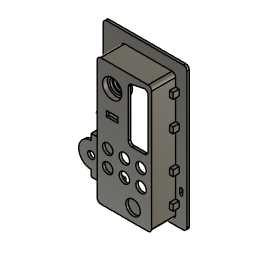
WIP-KV-1375DInputPanel-MULTIMOD (Autodesk Fusion 360 design; units mm, degrees)
Autodesk Fusion 360 part; units mm, degrees
sketch "Body" plane through (0, 0, 0) normal (0, 1, 0) x (1, 0, 0)
  line L0 (60.5, -7.2844) -> (60.5, -107.2844)
  circle A0 centre (0, -25.75) radius 10.5
  circle A1 centre (0, -25.75) radius 3
  arc A2 (18, -4.2844) -> (15, -7.2844) centre (18, -7.2844) ccw
  arc A3 (67, -119.5) -> (70, -116.5) centre (67, -116.5) ccw
  circle A4 centre (5.375, -59) radius 1
  line L1 (15, -4.2844) -> (19, -4.2844) construction
  line L2 (58.5105, -108.25) -> (17.001, -108.25)
  circle A5 centre (9.2756, -62.8749) radius 1
  arc A6 (57.5, -110.2844) -> (60.5, -107.2844) centre (57.5, -107.2844) ccw
  line L3 (0, -10) -> (0, -3)
  line L4 (15, -41.5) -> (0, -41.5)
  line L5 (15, -10) -> (15, -41.5)
  circle A7 centre (9.25, -59) radius 1.2
  arc A8 (15, -107.2844) -> (18, -110.2844) centre (18, -107.2844) ccw
  line L6 (70, -3) -> (70, -116.5)
  arc A9 (60.5, -7.2844) -> (57.5, -4.2844) centre (57.5, -7.2844) ccw
  line L7 (15, -107.2844) -> (15, -7.2844)
  arc A10 (70, -3) -> (67, 0) centre (67, -3) ccw
  circle A11 centre (9.25, -59) radius 3.875
  line L8 (17.0105, -6.25) -> (58.5105, -6.25)
  line L9 (18, -4.2844) -> (57.5, -4.2844)
  line L10 (0, -10) -> (15, -10)
  line L11 (3, 0) -> (67, 0)
  line L12 (67, -119.5) -> (3, -119.5)
  line L13 (57.5, -110.2844) -> (18, -110.2844)
  line L14 (58.5105, -6.25) -> (58.5105, -108.25)
  line L15 (0, -116.5) -> (0, -10)
  arc A12 (3, 0) -> (0, -3) centre (3, -3) ccw
  line L16 (15, -59) -> (9.25, -59)
  arc A13 (0, -116.5) -> (3, -119.5) centre (3, -116.5) ccw
  circle A14 centre (9.25, -55.125) radius 1
  line L17 (15, -100.2844) -> (12, -100.2844)
  line L18 (12, -100.2844) -> (12, -95.25)
  line L19 (12, -95.25) -> (15, -95.25)
  line L20 (15, -95.25) -> (15, -100.2844)
  line L21 (60.5, -100.2844) -> (63.5, -100.2844)
  line L22 (63.5, -100.2844) -> (63.5, -95.25)
  line L23 (63.5, -95.25) -> (60.5, -95.25)
  line L24 (60.5, -95.25) -> (60.5, -100.2844)
  line L25 (60.5, -75.25) -> (63.5, -75.25)
  line L26 (63.5, -75.25) -> (63.5, -70.25)
  line L27 (63.5, -70.25) -> (60.5, -70.25)
  line L28 (60.5, -70.25) -> (60.5, -75.25)
  line L29 (60.5, -44.25) -> (63.5, -44.25)
  line L30 (63.5, -44.25) -> (63.5, -39.25)
  line L31 (63.5, -39.25) -> (60.5, -39.25)
  line L32 (60.5, -39.25) -> (60.5, -44.25)
  line L33 (60.5, -14.2844) -> (63.5, -14.2844)
  line L34 (63.5, -14.2844) -> (63.5, -19.25)
  line L35 (63.5, -19.25) -> (60.5, -19.25)
  line L36 (60.5, -19.25) -> (60.5, -14.2844)
  line L37 (12.925, -58) -> (15, -58)
  line L38 (15, -58) -> (15, -60)
  line L39 (15, -60) -> (12.925, -60)
  line L40 (12.925, -60) -> (12.925, -58)
  line L41 (17.001, -108.25) -> (17.0105, -6.25)
  circle A15 centre (65.25, -28.5) radius 1.25
  circle A16 centre (65.25, -25) radius 1.25
  line L42 (65.25, -28.5) -> (64, -28.5)
  line L43 (65.25, -25) -> (66.5, -25)
  line L44 (64, -28.5) -> (66.5, -28.5)
  line L45 (66.5, -28.5) -> (66.5, -25)
  line L46 (66.5, -25) -> (64, -25)
  line L47 (64, -25) -> (64, -28.5)
  line L48 (15, -12) -> (0, -12)
  line L49 (15, -39.5) -> (0, -39.5)
  line L50 (15, -10) -> (17.0101, -10.0002)
  line L51 (15, -12) -> (17.0099, -12.0002)
  line L52 (15, -39.5) -> (17.0074, -39.5002)
  line L53 (15, -41.5) -> (17.0072, -41.5002)
  point P0 (54.389, -114.7651)
  point P1 (37.889, -114.7651)
  point P2 (70, 0)
  point P3 (0, -119.5)
  point P4 (60.5, -4.2844)
  point P5 (15, -110.2844)
  dimension "d245" = 70
  dimension "d246" = 119.5
  dimension "d247" = 45.5
  dimension "d248" = 106
  dimension "d249" = 31.5
  dimension "d250" = 21
  dimension "d251" = 6
  dimension "d252" = 5.75
  dimension "d253" = 2.4
  dimension "d254" = 7.75
  dimension "d256" = 2
  dimension "d257" = 2
  dimension "d258" = 2
  dimension "d260" = 41.5
  dimension "d261" = 102
  dimension "d262" = 3
  dimension "d263" = 3
  dimension "d484" = 10
  dimension "d485" = 10
  dimension "d486" = 10
  dimension "d487" = 20
  dimension "d488" = 20
  dimension "d757" = 2.5
  dimension "d758" = 2.5
  constraint horizontal L11
  constraint vertical L6
  constraint horizontal L12
  constraint horizontal L9
  constraint vertical L0
  constraint horizontal L13
  constraint vertical L7
  constraint horizontal L4
  constraint horizontal L10
  constraint vertical L5
  constraint coincident L4.start L7
  constraint concentric A0 A1
  constraint coincident L16.start L7
  constraint perpendicular L7 L16
  constraint coincident A7.centre A11.centre
  constraint coincident A5.centre A11
  constraint coincident A4.centre A11
  constraint coincident A14.centre A11
  constraint horizontal L1
  constraint horizontal L8
  constraint vertical L14
  constraint horizontal L2
  constraint perpendicular L10 L15
  constraint coincident L48.end L15
  constraint coincident L49.end L15
  constraint perpendicular L3 L11
  constraint coincident P3 L12
  constraint coincident P3 L15
  constraint tangent L12 A13
  constraint tangent L15 A13
  constraint tangent A3 L6
  constraint tangent A3 L12
  constraint equal A3 A13
  constraint coincident P2 L11
  constraint coincident P2 L6
  constraint tangent A10 L11
  constraint tangent L6 A10
  constraint equal A10 A13
  constraint coincident origin L11
  constraint tangent L3 A12
  constraint tangent L11 A12
  constraint equal A12 A13
  constraint coincident P5 L13
  constraint coincident P5 L7
  constraint tangent A8 L13
  constraint tangent A8 L7
  constraint tangent L0 A6
  constraint tangent A6 L13
  constraint equal A6 A8
  constraint coincident P4 L9
  constraint coincident P4 L0
  constraint tangent A9 L9
  constraint tangent L0 A9
  constraint equal A8 A9
  constraint coincident L1.start L7
  constraint coincident L1.start L9
  constraint tangent A2 L7
  constraint tangent A2 L9
  constraint equal A2 A8
  constraint horizontal L17
  constraint vertical L18
  constraint horizontal L19
  constraint vertical L20
  constraint coincident L7 L17.start
  constraint horizontal L21
  constraint vertical L22
  constraint horizontal L23
  constraint vertical L24
  constraint coincident L0 L21.start
  constraint horizontal L25
  constraint vertical L26
  constraint horizontal L27
  constraint vertical L28
  constraint coincident L0 L25.start
  constraint horizontal L29
  constraint vertical L30
  constraint horizontal L31
  constraint vertical L32
  constraint coincident L0 L29.start
  constraint horizontal L33
  constraint vertical L34
  constraint horizontal L35
  constraint vertical L36
  constraint coincident L0 L33.start
  constraint horizontal L37
  constraint vertical L38
  constraint horizontal L39
  constraint vertical L40
  constraint coincident L7 L38.end
  constraint coincident A15.centre L42.start
  constraint coincident A15 L42.end
  constraint horizontal L42
  constraint coincident A16.centre L43.start
  constraint coincident A16 L43.end
  constraint horizontal L43
  constraint horizontal L44
  constraint vertical L45
  constraint horizontal L46
  constraint vertical L47
  constraint coincident L5 L48.start
  constraint coincident L5 L49.start
  constraint coincident L41 L50.end
  constraint perpendicular L41 L50
  constraint coincident L41 L51.end
  constraint perpendicular L41 L51
  constraint coincident L41 L52.end
  constraint perpendicular L41 L52
  constraint coincident L41 L53.end
  constraint perpendicular L41 L53
  measures "d245" distance of origin P2
  measures "d246" distance of origin P3
  measures "d247" distance of L1.start P4
  measures "d248" distance of L1.start P5
  measures "d249" distance of L5.start L4.start
  measures "d250" diameter of A0
  measures "d251" diameter of A1
  measures "d252" distance of L16.start A7.centre
  measures "d253" diameter of A7
  measures "d254" diameter of A11
  measures "d256" diameter of A5
  measures "d257" diameter of A4
  measures "d258" diameter of A14
  measures "d260" distance of L8.start L8.end
  measures "d261" distance of L8.start L2.end
  measures "d262" radius of A13
  measures "d263" radius of A8
  measures "d484" distance of L13 L21
  measures "d485" distance of L9 L33
  measures "d486" distance of L13 L17
  measures "d487" distance of L31 L35
  measures "d488" distance of L23 L25
  measures "d757" diameter of A15
  measures "d758" diameter of A16
sketch "SCART" plane through (0, 0, 0) normal (0, 1, 0) x (1, 0, 0)
  line L0 (53.8762, -105.9949) -> (43.3762, -103.763)
  arc A0 (41, -100.8286) -> (43.3762, -103.763) centre (44, -100.8286) ccw
  arc A1 (53.8762, -105.9949) -> (57.5, -103.0604) centre (54.5, -103.0604) ccw
  arc A2 (44, -58.6151) -> (41, -61.6151) centre (44, -61.6151) ccw
  arc A3 (57.5, -61.6151) -> (54.5, -58.6151) centre (54.5, -61.6151) ccw
  line L1 (44, -56.6151) -> (55.389, -56.6151)
  line L2 (59.889, -61.6151) -> (59.889, -109.0604)
  line L3 (59.889, -109.0604) -> (39, -109.0604)
  line L4 (39, -109.0604) -> (39, -61.6151)
  arc A4 (44, -56.6151) -> (39, -61.6151) centre (44, -61.6151) ccw
  line L5 (59.889, -61.6151) -> (59.889, -56.6151)
  line L6 (59.889, -56.6151) -> (55.389, -56.6151)
  line L7 (41, -100.8286) -> (41, -61.6151)
  line L8 (44, -58.6151) -> (54.5, -58.6151)
  line L9 (57.5, -61.6151) -> (57.5, -103.0604)
  dimension "d178" = 3
  dimension "d179" = 3
  dimension "d180" = 3
  dimension "d181" = 3
  dimension "d183" = 39.2135
  constraint tangent L0 A1
  constraint tangent L0 A0
  constraint horizontal L1
  constraint vertical L2
  constraint horizontal L3
  constraint vertical L4
  constraint tangent L1 A4
  constraint tangent L4 A4
  constraint perpendicular L1 L5
  constraint perpendicular L5 L6
  constraint tangent A2 L7
  constraint tangent A3 L8
  constraint tangent A1 L9
  measures "d178" radius of A1
  measures "d179" radius of A0
  measures "d180" radius of A2
  measures "d181" radius of A3
  measures "d183" distance of A2.end A0.start
sketch "Components" plane through (0, 0, 0) normal (0, 1, 0) x (1, 0, 0)
  circle A0 centre (37.705, -33.2295) radius 5.75
  circle A1 centre (37.705, -33.2295) radius 6.5
  circle A2 centre (23.805, -33.2295) radius 6.5
  circle A3 centre (23.805, -33.2295) radius 5.75
  circle A4 centre (51.605, -33.2295) radius 5.75
  circle A5 centre (51.605, -33.2295) radius 6.5
  circle A6 centre (37.705, -33.2295) radius 4.375
  circle A7 centre (23.805, -33.2295) radius 4.375
  circle A8 centre (51.605, -33.2295) radius 4.375
  circle A9 centre (51.605, -47.1295) radius 6.5
  circle A10 centre (37.705, -47.1295) radius 5.75
  circle A11 centre (51.605, -47.1295) radius 5.75
  circle A12 centre (37.705, -47.1295) radius 6.5
  circle A13 centre (23.805, -47.1295) radius 5.75
  circle A14 centre (37.705, -47.1295) radius 4.375
  circle A15 centre (51.605, -47.1295) radius 4.375
  circle A16 centre (23.805, -47.1295) radius 6.5
  circle A17 centre (23.805, -47.1295) radius 4.375
  circle A18 centre (27.5005, -92.5463) radius 4.825
  circle A19 centre (27.5005, -92.5463) radius 9
  circle A20 centre (27.5005, -92.5463) radius 8
  line L0 (19.5004, -75.9605) -> (35.5004, -75.9605)
  line L1 (22.7504, -74.4605) -> (22.7504, -69.9605)
  line L2 (19.5004, -68.4605) -> (19.5004, -75.9605)
  line L3 (32.2504, -69.9605) -> (32.2504, -74.4605)
  line L4 (22.7504, -69.9605) -> (32.2504, -69.9605)
  line L5 (32.2504, -74.4605) -> (22.7504, -74.4605)
  line L6 (33.2504, -75.4605) -> (33.2504, -68.9605)
  line L7 (21.7504, -68.9605) -> (21.7504, -75.4605)
  line L8 (33.2504, -68.9605) -> (21.7504, -68.9605)
  line L9 (35.5004, -68.4605) -> (19.5004, -68.4605)
  line L10 (15.5004, -77.9605) -> (15.5004, -66.4605)
  line L11 (38.5004, -66.4605) -> (38.5004, -77.9605)
  line L12 (35.5004, -75.9605) -> (35.5004, -68.4605)
  line L13 (21.7504, -75.4605) -> (33.2504, -75.4605)
  line L14 (15.5004, -66.4605) -> (38.5004, -66.4605)
  line L15 (38.5004, -77.9605) -> (15.5004, -77.9605)
  circle A21 centre (55.0033, -15.1761) radius 1.25
  circle A22 centre (35.0033, -15.1761) radius 1.25
  circle A23 centre (45.0033, -15.1761) radius 6.125
  line L16 (21.9579, -89.347) -> (21.958, -95.747)
  line L17 (27.5008, -98.9466) -> (33.0434, -95.7468)
  line L18 (27.5003, -86.1467) -> (21.9579, -89.347)
  line L19 (33.0434, -95.7468) -> (33.0428, -89.3468)
  line L20 (33.0428, -89.3468) -> (27.5003, -86.1467)
  line L21 (21.958, -95.747) -> (27.5008, -98.9466)
  line L22 (51.605, -47.1295) -> (51.605, -33.2295)
  line L23 (23.805, -33.2295) -> (23.805, -47.1295)
  line L24 (37.705, -47.1295) -> (37.705, -33.2295)
  line L25 (23.805, -47.1295) -> (37.705, -47.1295)
  line L26 (37.705, -47.1295) -> (51.605, -47.1295)
  line L27 (30.755, -47.1295) -> (30.755, -33.7)
  line L28 (44.655, -47.1295) -> (44.655, -33.7)
  circle A24 centre (30.755, -40.1795) radius 1.25
  circle A25 centre (44.655, -40.1795) radius 1.25
  circle A26 centre (55.0033, -15.1761) radius 2.93
  circle A27 centre (35.0033, -15.1761) radius 2.9
  circle A28 centre (45.0033, -15.1761) radius 6.85
  line L29 (56.0709, -17.9047) -> (48.0733, -21.2996)
  line L30 (56.0709, -12.4476) -> (48.0733, -9.0526)
  line L31 (34.0209, -17.9047) -> (41.9332, -21.2996)
  line L32 (34.0209, -12.4476) -> (41.9332, -9.0526)
  circle A29 centre (27.5005, -92.5463) radius 6
  line L33 (24.6242, -97.8165) -> (30.3742, -97.8165)
  line L34 (44.655, -33.7) -> (45.1221, -33.7)
  line L35 (44.655, -33.7) -> (44.188, -33.7)
  line L36 (30.755, -33.7) -> (31.2221, -33.7)
  line L37 (30.755, -33.7) -> (30.288, -33.7)
  point P0 (37.889, -53.1151)
  point P1 (27.5005, -92.5463)
  dimension "d301" = 8.75
  dimension "d302" = 8.75
  dimension "d303" = 8.75
  dimension "d304" = 11.5
  dimension "d305" = 11.5
  dimension "d306" = 11.5
  dimension "d307" = 13
  dimension "d308" = 13
  dimension "d309" = 13
  dimension "d334" = 13.9
  dimension "d384" = 8.75
  dimension "d385" = 8.75
  dimension "d386" = 8.75
  dimension "d387" = 11.5
  dimension "d388" = 11.5
  dimension "d389" = 11.5
  dimension "d390" = 13
  dimension "d391" = 13
  dimension "d392" = 13
  dimension "d393" = 13.9
  dimension "d395" = 13.9
  dimension "d400" = 9.65
  dimension "d401" = 16
  dimension "d402" = 18
  dimension "d403" = 7.5
  dimension "d404" = 16
  dimension "d405" = 4.5
  dimension "d406" = 9.5
  dimension "d407" = 6.5
  dimension "d408" = 11.5
  dimension "d409" = 7.5
  dimension "d410" = 16
  dimension "d411" = 11.5
  dimension "d412" = 6.5
  dimension "d413" = 4.5
  dimension "d414" = 2.25
  dimension "d415" = 2.25
  dimension "d416" = 1
  dimension "d417" = 12.25
  dimension "d420" = 2.5
  dimension "d422" = 2.5
  dimension "d787" = 13.9
  dimension "d788" = 13.9
  dimension "d791" = 2.5
  dimension "d792" = 2.5
  dimension "d793" = 13.9
  dimension "d805" = 5.86
  dimension "d806" = 5.8
  dimension "d807" = 13.7
  dimension "d818" = 3
  dimension "d851" = 12
  dimension "d852" = 5.75
  constraint concentric A3 A7
  constraint concentric A0 A6
  constraint concentric A4 A8
  constraint concentric A2 A3
  constraint concentric A1 A6
  constraint concentric A5 A8
  constraint concentric A13 A17
  constraint concentric A10 A14
  constraint concentric A11 A15
  constraint concentric A13 A16
  constraint concentric A12 A14
  constraint concentric A9 A15
  constraint concentric A18 A20
  constraint concentric A18 A19
  constraint perpendicular L1 L4
  constraint perpendicular L7 L8
  constraint perpendicular L2 L9
  constraint perpendicular L0 L12
  constraint perpendicular L3 L5
  constraint horizontal L15
  constraint vertical L10
  constraint horizontal L14
  constraint vertical L11
  constraint vertical L22
  constraint vertical L23
  constraint coincident A4.centre A5.centre
  constraint coincident A13.centre A16.centre
  constraint coincident A10.centre A12.centre
  constraint coincident A0.centre A1.centre
  constraint perpendicular L24 L25
  constraint coincident A9.centre A11.centre
  constraint perpendicular L22 L26
  constraint midpoint L25 L27.start
  constraint perpendicular L25 L27
  constraint midpoint L26 L28.start
  constraint perpendicular L26 L28
  constraint coincident L27 A24.centre
  constraint coincident L28 A25.centre
  constraint concentric A21 A26
  constraint concentric A22 A27
  constraint coincident A26 L29.start
  constraint coincident A28 L29.end
  constraint coincident A26 L30.start
  constraint coincident A28 L30.end
  constraint coincident A28 L32.end
  constraint coincident A28 L31.end
  constraint coincident A27 L31.start
  constraint coincident A27 L32.start
  constraint coincident P1 A18.centre
  constraint horizontal L33
  constraint coincident A5 L34.end
  constraint perpendicular L28 L34
  constraint coincident A1 L35.end
  constraint perpendicular L28 L35
  constraint coincident A1 L36.end
  constraint perpendicular L27 L36
  constraint coincident A2 L37.end
  constraint perpendicular L27 L37
  measures "d301" diameter of A7
  measures "d302" diameter of A6
  measures "d303" diameter of A8
  measures "d304" diameter of A3
  measures "d305" diameter of A0
  measures "d306" diameter of A4
  measures "d307" diameter of A2
  measures "d308" diameter of A1
  measures "d309" diameter of A5
  measures "d334" distance of A4.centre A0.centre
  measures "d384" diameter of A17
  measures "d385" diameter of A14
  measures "d386" diameter of A15
  measures "d387" diameter of A13
  measures "d388" diameter of A10
  measures "d389" diameter of A11
  measures "d390" diameter of A16
  measures "d391" diameter of A12
  measures "d392" diameter of A9
  measures "d393" distance of A10.centre A9.centre
  measures "d395" distance of A2.centre A13.centre
  measures "d400" diameter of A18
  measures "d401" diameter of A20
  measures "d402" diameter of A19
  measures "d403" distance of L2.start L0.start
  measures "d404" distance of L2.start L9.start
  measures "d405" distance of L1.start L1.end
  measures "d406" distance of L3.start L1.end
  measures "d407" distance of L7.end L7.start
  measures "d408" distance of L6.end L7.start
  measures "d409" vertical distance of L0.end L9.start
  measures "d410" distance of L0.end L0.start
  measures "d411" distance of L7.end L6.start
  measures "d412" distance of L6.end L6.start
  measures "d413" distance of L3.start L3.end
  measures "d414" distance of L2 L7
  measures "d415" distance of L6 L12
  measures "d416" distance of L1 L7
  measures "d417" diameter of A23
  measures "d420" diameter of A22
  measures "d422" diameter of A21
  measures "d787" distance of A0.centre A2.centre
  measures "d788" distance of A10.centre A13.centre
  measures "d791" diameter of A24
  measures "d792" diameter of A25
  measures "d793" distance of A24.centre A25.centre
  measures "d805" diameter of A26
  measures "d806" diameter of A27
  measures "d807" diameter of A28
  measures "d818" distance of L11 L12
  measures "d851" diameter of A29
  measures "d852" distance of L33.start L33.end
sketch "Text" plane through (0, 0, 0) normal (0, 1, 0) x (1, 0, 0)
  line L0 (21.7063, -54.3471) -> (24.4568, -54.3477) construction
  line L1 (24.4568, -54.3477) -> (24.4559, -58.6235) construction
  line L2 (24.4559, -58.6235) -> (21.7054, -58.623) construction
  line L3 (21.7054, -58.623) -> (21.7063, -54.3471) construction
  line L4 (36.3063, -54.3471) -> (39.0568, -54.3477) construction
  line L5 (39.0568, -54.3477) -> (39.0559, -58.6235) construction
  line L6 (39.0559, -58.6235) -> (36.3054, -58.623) construction
  line L7 (36.3054, -58.623) -> (36.3063, -54.3471) construction
  line L8 (50.9063, -54.3471) -> (53.6568, -54.3477) construction
  line L9 (53.6568, -54.3477) -> (53.6559, -58.6235) construction
  line L10 (53.6559, -58.6235) -> (50.9054, -58.623) construction
  line L11 (50.9054, -58.623) -> (50.9063, -54.3471) construction
  line L12 (21.7063, -21.9471) -> (24.4568, -21.9477) construction
  line L13 (24.4568, -21.9477) -> (24.4559, -26.2235) construction
  line L14 (24.4559, -26.2235) -> (21.7054, -26.223) construction
  line L15 (21.7054, -26.223) -> (21.7063, -21.9471) construction
  line L16 (34.3063, -21.9471) -> (37.0568, -21.9477) construction
  line L17 (37.0568, -21.9477) -> (37.0559, -26.2235) construction
  line L18 (37.0559, -26.2235) -> (34.3054, -26.223) construction
  line L19 (34.3054, -26.223) -> (34.3063, -21.9471) construction
  line L20 (52.9063, -21.9471) -> (55.6568, -21.9477) construction
  line L21 (55.6568, -21.9477) -> (55.6559, -26.2235) construction
  line L22 (55.6559, -26.2235) -> (52.9054, -26.223) construction
  line L23 (52.9054, -26.223) -> (52.9063, -21.9471) construction
  line L24 (34.3059, -21.947) -> (55.6564, -21.9476) construction
  line L25 (55.6564, -21.9476) -> (55.6563, -26.2236) construction
  line L26 (55.6563, -26.2236) -> (34.3058, -26.223) construction
  line L27 (34.3058, -26.223) -> (34.3059, -21.947) construction
  line L28 (24.679, -76.0314) -> (37.8631, -76.041) construction
  line L29 (37.8631, -76.041) -> (37.86, -80.3168) construction
  line L30 (37.86, -80.3168) -> (24.6759, -80.3072) construction
  line L31 (24.6759, -80.3072) -> (24.679, -76.0314) construction
  line L32 (16.8252, -103.6603) -> (38.0757, -103.6645) construction
  line L33 (38.0757, -103.6645) -> (38.0749, -107.9404) construction
  line L34 (38.0749, -107.9404) -> (16.8244, -107.9361) construction
  line L35 (16.8244, -107.9361) -> (16.8252, -103.6603) construction
  line L36 (17.4025, -13.5113) -> (24.4026, -13.5124) construction
  line L37 (24.4026, -13.5124) -> (24.4022, -15.7884) construction
  line L38 (24.4022, -15.7884) -> (17.4021, -15.7872) construction
  line L39 (17.4021, -15.7872) -> (17.4025, -13.5113) construction
  line L40 (15.8532, -62.6768) -> (24.6037, -62.6786) construction
  line L41 (24.6037, -62.6786) -> (24.6029, -66.9544) construction
  line L42 (24.6029, -66.9544) -> (15.8523, -66.9527) construction
  line L43 (15.8523, -66.9527) -> (15.8532, -62.6768) construction
  line L44 (30.3533, -62.1768) -> (39.1038, -62.1786) construction
  line L45 (39.1038, -62.1786) -> (39.1029, -66.9544) construction
  line L46 (39.1029, -66.9544) -> (30.3523, -66.9527) construction
  line L47 (30.3523, -66.9527) -> (30.3533, -62.1768) construction
  circle A0 centre (45.0033, -15.1761) radius 6.125
  line L48 (17.0051, -76.0235) -> (24.6796, -76.0314) construction
  line L49 (24.6796, -76.0314) -> (24.6752, -80.3072) construction
  line L50 (24.6752, -80.3072) -> (17.0007, -80.2994) construction
  line L51 (17.0007, -80.2994) -> (17.0051, -76.0235) construction
  line L52 (24.4026, -13.5125) -> (31.153, -13.5139) construction
  line L53 (31.153, -13.5139) -> (31.1526, -15.7897) construction
  line L54 (31.1526, -15.7897) -> (24.4022, -15.7883) construction
  line L55 (24.4022, -15.7883) -> (24.4026, -13.5125) construction
  point P0 (23.805, -47.1295)
  dimension "d444" = 2.5
  dimension "d449" = 2.5
  dimension "d450" = 2.5
  dimension "d459" = 2.5
  dimension "d460" = 2.5
  dimension "d461" = 2.5
  dimension "d462" = 2.25
  dimension "d463" = 2.25
  dimension "d464" = 2.5
  dimension "d465" = 2.5
  dimension "d480" = 2
  dimension "d481" = 2
  dimension "d773" = 2.5
  dimension "d774" = 2.25
  constraint midpoint L21
  constraint midpoint L19
  constraint midpoint L55
sketch "Detail" plane through (0, 0, 0) normal (0, 1, 0) x (1, 0, 0)
  line L0 (22.7504, -74.4605) -> (22.7504, -69.9605)
  line L1 (20.056, -71.0355) -> (20.056, -69)
  line L2 (20.056, -69) -> (19.306, -69)
  line L3 (22.7504, -72.2105) -> (22.7504, -72.5855)
  line L4 (22.7504, -72.5855) -> (20.806, -72.5855)
  line L5 (19.306, -71.0855) -> (19.306, -69)
  line L6 (22.7504, -72.2105) -> (22.7504, -71.8355)
  line L7 (22.7504, -71.8355) -> (20.856, -71.8355)
  line L8 (32.2504, -74.4605) -> (22.7504, -74.4605)
  line L9 (22.7504, -69.9605) -> (32.2504, -69.9605)
  line L10 (27.5004, -74.4605) -> (27.5004, -69.9605)
  line L11 (32.2504, -72.5855) -> (34.1948, -72.5855)
  line L12 (32.2504, -72.2105) -> (32.2504, -71.8355)
  line L13 (32.2504, -72.2105) -> (32.2504, -72.5855)
  line L14 (32.2504, -71.8355) -> (34.1448, -71.8355)
  line L15 (34.9448, -71.0355) -> (34.9448, -69)
  line L16 (35.6948, -71.0855) -> (35.6948, -69)
  line L17 (34.9448, -69) -> (35.6948, -69)
  circle A0 centre (19.681, -69) radius 0.375
  circle A1 centre (35.3198, -69) radius 0.375
  arc A2 (20.056, -71.0355) -> (20.856, -71.8355) centre (20.856, -71.0355) ccw
  arc A3 (19.306, -71.0855) -> (20.806, -72.5855) centre (20.806, -71.0855) ccw
  arc A4 (34.1448, -71.8355) -> (34.9448, -71.0355) centre (34.1448, -71.0355) ccw
  arc A5 (34.1948, -72.5855) -> (35.6948, -71.0855) centre (34.1948, -71.0855) ccw
  line L18 (21.5279, -39.1717) -> (26.0988, -39.1717)
  line L19 (29.7556, -35.5149) -> (29.7556, -30.944)
  line L20 (26.0988, -27.2873) -> (21.5279, -27.2873)
  line L21 (17.8712, -30.944) -> (17.8712, -35.5149)
  line L22 (21.5279, -39.8573) -> (26.0988, -39.8573)
  line L23 (30.4412, -35.5149) -> (30.4412, -30.944)
  line L24 (26.0988, -26.6016) -> (21.5279, -26.6016)
  line L25 (17.1855, -30.944) -> (17.1855, -35.5149)
  arc A6 (17.8712, -35.5149) -> (21.5279, -39.1717) centre (21.5279, -35.5149) ccw
  arc A7 (21.5279, -27.2873) -> (17.8712, -30.944) centre (21.5279, -30.944) ccw
  arc A8 (29.7556, -30.944) -> (26.0988, -27.2873) centre (26.0988, -30.944) ccw
  arc A9 (26.0988, -39.1717) -> (29.7556, -35.5149) centre (26.0988, -35.5149) ccw
  arc A10 (17.1855, -35.5149) -> (21.5279, -39.8573) centre (21.5279, -35.5149) ccw
  arc A11 (26.0988, -39.8573) -> (30.4412, -35.5149) centre (26.0988, -35.5149) ccw
  arc A12 (21.5279, -26.6016) -> (17.1855, -30.944) centre (21.5279, -30.944) ccw
  arc A13 (30.4412, -30.944) -> (26.0988, -26.6016) centre (26.0988, -30.944) ccw
  circle A14 centre (45.0033, -15.1761) radius 6.625
  circle A15 centre (45.0033, -15.1761) radius 7.375
  line L26 (33.9, -15.5511) -> (38.3889, -15.5511)
  line L27 (38.3889, -15.5511) -> (38.3889, -14.8011)
  line L28 (38.3889, -14.8011) -> (33.9, -14.8011)
  line L29 (33.9, -14.8011) -> (33.9, -15.5511)
  circle A16 centre (33.9, -15.1761) radius 0.375
  line L30 (21.7504, -72.5855) -> (21.7504, -71.8355)
  line L31 (33.2504, -72.5855) -> (33.2504, -71.8355)
  line L32 (21.0561, -71.8355) -> (21.0561, -72.6)
  line L33 (33.9447, -71.8355) -> (33.9447, -72.6)
  line L34 (31.0755, -30.944) -> (31.0755, -35.5149)
  arc A17 (31.7612, -35.5149) -> (35.4179, -39.1717) centre (35.4179, -35.5149) ccw
  arc A18 (35.4179, -27.2873) -> (31.7612, -30.944) centre (35.4179, -30.944) ccw
  line L35 (31.7612, -30.944) -> (31.7612, -35.5149)
  arc A19 (31.0755, -35.5149) -> (35.4179, -39.8573) centre (35.4179, -35.5149) ccw
  arc A20 (35.4179, -26.6016) -> (31.0755, -30.944) centre (35.4179, -30.944) ccw
  line L36 (57.5356, -35.5149) -> (57.5356, -30.944)
  arc A21 (58.2212, -30.944) -> (53.8788, -26.6016) centre (53.8788, -30.944) ccw
  arc A22 (53.8788, -39.1717) -> (57.5356, -35.5149) centre (53.8788, -35.5149) ccw
  arc A23 (53.8788, -39.8573) -> (58.2212, -35.5149) centre (53.8788, -35.5149) ccw
  line L37 (58.2212, -35.5149) -> (58.2212, -30.944)
  arc A24 (57.5356, -30.944) -> (53.8788, -27.2873) centre (53.8788, -30.944) ccw
  arc A25 (53.8788, -53.0617) -> (57.5356, -49.4049) centre (53.8788, -49.4049) ccw
  line L38 (58.2212, -49.4049) -> (58.2212, -44.834)
  arc A26 (58.2212, -44.834) -> (53.8788, -40.4916) centre (53.8788, -44.834) ccw
  line L39 (57.5356, -49.4049) -> (57.5356, -44.834)
  arc A27 (17.8712, -49.4049) -> (21.5279, -53.0617) centre (21.5279, -49.4049) ccw
  arc A28 (57.5356, -44.834) -> (53.8788, -41.1773) centre (53.8788, -44.834) ccw
  arc A29 (21.5279, -41.1773) -> (17.8712, -44.834) centre (21.5279, -44.834) ccw
  arc A30 (53.8788, -53.7473) -> (58.2212, -49.4049) centre (53.8788, -49.4049) ccw
  line L40 (17.1855, -44.834) -> (17.1855, -49.4049)
  arc A31 (17.1855, -49.4049) -> (21.5279, -53.7473) centre (21.5279, -49.4049) ccw
  arc A32 (21.5279, -40.4916) -> (17.1855, -44.834) centre (21.5279, -44.834) ccw
  line L41 (17.8712, -44.834) -> (17.8712, -49.4049)
  line L42 (21.5279, -53.7473) -> (53.8788, -53.7473)
  line L43 (21.5279, -53.0617) -> (53.8788, -53.0617)
  line L44 (21.5279, -41.1773) -> (53.8788, -41.1773)
  line L45 (21.5279, -40.4916) -> (53.8788, -40.4916)
  line L46 (35.4179, -39.8573) -> (53.8788, -39.8573)
  line L47 (35.4179, -39.1717) -> (53.8788, -39.1717)
  line L48 (35.4179, -27.2873) -> (53.8788, -27.2873)
  line L49 (35.4179, -26.6016) -> (53.8788, -26.6016)
  point P0 (45.0033, -15.1761)
  dimension "d563" = 0.75
  dimension "d564" = 0.75
  dimension "d565" = 0.8
  dimension "d566" = 1.5
  dimension "d567" = 0.8
  dimension "d568" = 1.5
  dimension "d620" = 13.25
  dimension "d621" = 14.75
  dimension "d624" = 0.75
  constraint midpoint L0 L3.start
  constraint perpendicular L1 L2
  constraint perpendicular L3 L4
  constraint perpendicular L2 L5
  constraint perpendicular L1 L7
  constraint midpoint L8 L10.start
  constraint midpoint L9 L10.end
  constraint symmetric L3.start L10 L12.start
  constraint symmetric L1.end L10 L15.end
  constraint symmetric L2.end L10 L16.end
  constraint symmetric L3.end L10 L11.start
  constraint symmetric L6.end L10 L12.end
  constraint midpoint L2 A0.centre
  constraint midpoint L17 A1.centre
  constraint tangent L1 A2
  constraint tangent L7 A2
  constraint tangent L4 A3
  constraint tangent L5 A3
  constraint tangent L14 A4
  constraint tangent L15 A4
  constraint tangent L11 A5
  constraint tangent L16 A5
  constraint horizontal L18
  constraint vertical L19
  constraint horizontal L20
  constraint vertical L21
  constraint horizontal L24
  constraint vertical L25
  constraint tangent L18 A6
  constraint tangent L21 A6
  constraint tangent L20 A7
  constraint tangent L21 A7
  constraint tangent L19 A8
  constraint tangent L20 A8
  constraint tangent L18 A9
  constraint tangent L19 A9
  constraint tangent L25 A10
  constraint tangent L23 A11
  constraint tangent L24 A12
  constraint tangent L25 A12
  constraint tangent L23 A13
  constraint tangent L24 A13
  constraint coincident P0 A14.centre
  constraint concentric A14 A15
  constraint horizontal L26
  constraint vertical L27
  constraint horizontal L28
  constraint vertical L29
  constraint coincident A14 L27.end
  constraint midpoint L29 A16.centre
  constraint coincident L4 L30.start
  constraint coincident L7 L30.end
  constraint perpendicular L7 L30
  constraint coincident L11 L31.start
  constraint coincident L14 L31.end
  constraint perpendicular L14 L31
  constraint coincident L7 L32.start
  constraint perpendicular L7 L32
  constraint symmetric L10 L32.start L33.start
  constraint symmetric L10 L32.end L33.end
  constraint vertical L35
  constraint vertical L34
  constraint tangent A17 L35
  constraint tangent A18 L35
  constraint tangent L34 A19
  constraint tangent L34 A20
  constraint vertical L36
  constraint tangent L36 A24
  constraint tangent L36 A22
  constraint tangent A23 L37
  constraint tangent A21 L37
  constraint vertical L41
  constraint vertical L40
  constraint tangent A27 L41
  constraint tangent A29 L41
  constraint tangent L40 A31
  constraint tangent L40 A32
  constraint vertical L39
  constraint tangent L39 A28
  constraint tangent A25 L39
  constraint tangent L38 A30
  constraint tangent L38 A26
  constraint tangent A30 L42
  constraint tangent A25 L43
  constraint tangent A28 L44
  constraint tangent A26 L45
  constraint tangent A23 L46
  constraint tangent A22 L47
  constraint tangent A18 L48
  constraint tangent A21 L49
  measures "d563" diameter of A0
  measures "d564" diameter of A1
  measures "d565" radius of A2
  measures "d566" radius of A3
  measures "d567" radius of A4
  measures "d568" radius of A5
  measures "d620" diameter of A14
  measures "d621" diameter of A15
  measures "d624" diameter of A16
extrude "Extrude89" cut sketch "Components" against normal blind 1 contours A21 | A22
move_body "Move28" [no effect]
move_body "Move30" [no effect]
extrude "Extrude103" cut sketch "Components" sketch "SCART" along normal blind 2 contours A0 | A10 A14 L24 L25 | A10 A14 L24 L26 | A10 A14 L25 L26 | A14 L24 L25 | A14 L24 L26 | A14 L25 L26 | A13 A17 L23 L25 | A13 A17 L23 L25 | A11 A15 L22 L26 | A11 A15 L22 L26 | A17 L23 L25 | A17 L23 L25 | A15 L22 L26 | A15 L22 L26 | A3 | A4 | A6 | A7 | A8 | A18 | A20 | L1 L3 L4 L5 | A23 | L16 L18 A29 | L16 L17 L18 L19 L20 L21 A29 L33 | L16 A29 | L18 A29 | L16 L21 A29 | L18 L20 A29 | L21 A29 L33 | L20 A29 | L17 L21 A29 L33 | L21 A29 L33 | L19 L20 A29 | L17 L21 A29 | L17 A29 L33 | L17 A29 L33 | L19 A29 | L17 L19 A29 of sketch 2 contours L0 A0 A1 A2 A3 L7 L8 L9
extrude "Extrude134" add sketch "Body" along normal blind 2 separate body contours L0 A2 L2 A6 A8 A9 L7 L8 L9 L13 L14 L20 L24 L28 L32 L36 L38 L41 L50 L53 | L5 L7 L41 L50 L51 | L5 L7 L41 L51 L52 | L2 L8 L14 L41 | L5 L7 L41 L52 L53 makes body 1
move_body "Move51" bodies 1 to x (1, 0, 0) y (0, 1, 0) z (0, 0, 1) at (0, -2, 0)
extrude "Extrude135" add sketch "Body" along normal blind 18 contours L0 A2 L2 A6 A8 A9 L7 L8 L9 L13 L14 L20 L24 L28 L32 L36 L38 L41 L50 L53 | L5 L7 L41 L50 L51 | L5 L7 L41 L52 L53 bodies 1
extrude "Extrude136" add sketch "Body" along normal blind 10 contours L5 L7 L41 L51 L52 bodies 1
move_body "Move52" bodies 1 to x (1, 0, 0) y (0, 1, 0) z (0, 0, 1) at (0, -8, 0)
extrude "Extrude137" add sketch "Body" along normal blind 2 contours L5 L7 L10 L15 L48 | A0 L5 L7 L15 L48 L49 | L4 L5 L7 L15 L49 | A0 A1 L15 | A0 A1 L15 bodies 1
extrude "Extrude138" add sketch "Body" along normal blind 10 contours L5 L7 L10 L15 L48 | L4 L5 L7 L15 L49 bodies 1
move_body "Move53" bodies 1 to x (1, 0, 0) y (0, 1, 0) z (0, 0, 1) at (0, -10, 0)
extrude "Extrude139" add sketch "Body" along normal blind 2 contours L0 A2 A3 A4 A5 A6 L3 L4 A8 L6 A9 L7 A10 A11 L9 L10 L11 L12 L13 L15 A12 A13 A14 L17 L18 L19 L21 L22 L23 L25 L26 L27 L29 L30 L31 L33 L34 L35 L37 L39 | L0 A2 L2 A6 A8 A9 L7 L8 L9 L13 L14 L20 L24 L28 L32 L36 L38 L41 L50 L53 | L0 L33 L34 L35 L36 | L0 L29 L30 L31 L32 | L5 L7 L41 L50 L51 | L5 L7 L10 L15 L48 | L0 L25 L26 L27 L28 | L5 L7 L41 L52 L53 | L4 L5 L7 L15 L49 | L0 L21 L22 L23 L24 | L7 A11 L16 L37 L38 | L7 A11 L16 L38 L39 | A4 A5 A11 A14 L37 L39 L40 | A11 L16 L37 L40 | A11 L16 L39 L40 | A11 A14 | A11 A14 | L7 L17 L18 L19 L20 | A5 A11 | A5 A11 | A4 A11 | A4 A11 | A7 bodies 1
extrude "Extrude140" add sketch "Body" against normal blind 5 contours L0 L33 L34 L35 L36 | L0 L29 L30 L31 L32 | L0 L25 L26 L27 L28 | L0 L21 L22 L23 L24 | L7 L17 L18 L19 L20 bodies 1
extrude "Extrude141" add sketch "Body" against normal blind 10 contours L7 A11 L16 L37 L38 | L7 A11 L16 L38 L39 | A4 A5 A11 A14 L37 L39 L40 | A11 L16 L37 L40 | A11 L16 L39 L40 | A11 A14 | A11 A14 | A5 A11 | A5 A11 | A4 A11 | A4 A11 bodies 1
move_body "Move54" bodies 1 to x (1, 0, 0) y (0, 1, 0) z (0, 0, 1) at (0, 20, 0)
extrude "Extrude142" cut sketch "Components" sketch "SCART" sketch "Text" along normal blind 2 contours A14 L24 L25 | A14 L24 L26 | A14 L25 L26 | A17 L23 L25 | A17 L23 L25 | A15 L22 L26 | A15 L22 L26 | A6 | A7 | A8 | A18 | L1 L3 L4 L5 of sketch 2 contours L0 A0 A1 A2 A3 L7 L8 L9 of sketch 3 bodies 1
extrude "Extrude143" add sketch "Components" along normal blind 8 contours A19 | A20 | L16 L18 A29 | L16 L17 L18 L19 L20 L21 A29 L33 | L16 A29 | L18 A29 | L16 L21 A29 | L18 L20 A29 | L21 A29 L33 | L20 A29 | L17 L21 A29 L33 | L21 A29 L33 | L19 L20 A29 | L17 L21 A29 | L17 A29 L33 | L17 A29 L33 | L19 A29 | L17 L19 A29 bodies 1
extrude "Extrude144" cut sketch "Components" along normal blind 6 contours A19 | A20 | L16 L18 A29 | L16 L17 L18 L19 L20 L21 A29 L33 | L16 A29 | L18 A29 | L16 L21 A29 | L18 L20 A29 | L21 A29 L33 | L20 A29 | L17 L21 A29 L33 | L21 A29 L33 | L19 L20 A29 | L17 L21 A29 | L17 A29 L33 | L17 A29 L33 | L19 A29 | L17 L19 A29 bodies 1 makes body 2 at (35.0573, 6, 93.2332)
extrude "Extrude145" add sketch "Components" along normal blind 6 contours A19 bodies 1 2
extrude "Extrude146" add sketch "Components" along normal blind 6 contours A20 | L16 L18 A29 | L16 L21 A29 | L18 L20 A29 | L17 L21 A29 L33 | L21 A29 L33 | L19 L20 A29 | L17 L21 A29 | L17 A29 L33 | L17 L19 A29 picked at (25.6129, -98.0997) picked at (29.3884, -98.0996) bodies 1
extrude "Extrude147" cut sketch "Components" along normal blind 4 contours A20 | L16 L18 A29 | L16 L21 A29 | L18 L20 A29 | L17 L21 A29 L33 | L21 A29 L33 | L19 L20 A29 | L17 L21 A29 | L17 A29 L33 | L17 L19 A29 picked at (25.6129, -98.0997) picked at (29.3884, -98.0996) bodies 1
move_body "Move55" bodies 1 to x (1, 0, 0) y (0, 1, 0) z (0, 0, 1) at (0, -8, 0)
extrude "Extrude148" cut sketch "Components" against normal blind 1 contours L16 L18 A29 | L16 L17 L18 L19 L20 L21 A29 L33 | L16 L21 A29 | L18 L20 A29 | L17 L21 A29 L33 | L19 L20 A29 | L17 L21 A29 | L17 L19 A29 bodies 1
extrude "Extrude149" add 1 faces at (30.1524, -1, 97.1394) along direction (0, 1, 0) blind 1 on bodies 1 bodies 1
equation "d417 = 11.9 mm + 0.35 mm"
